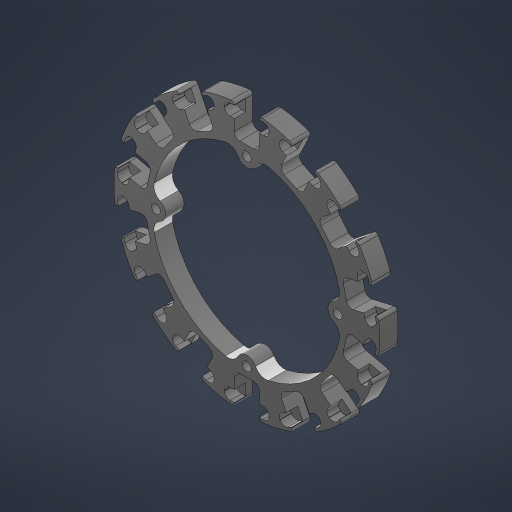
# Autodesk Inventor part: Wheel_Flame
Saved by Autodesk Inventor 2024.2 (Build 282272000, 272)
## iProperties
Created: 2023-12-20
Part Number: Wheel_Flame
Material: 一般
Document SubType Name: Modeling
Designer: Hanaoka
Density: 1 g/cm^3
Appearance: 黒
Author: Hanaoka
Autodesk Inventor part; units mm, degrees
ref_plane "YZ Plane" through (0, 0, 0) normal (1, 0, 0) x (0, 1, 0)
ref_plane "XZ Plane" through (0, 0, 0) normal (0, 1, 0) x (-1, 0, 0)
ref_plane "XY Plane" through (0, 0, 0) normal (0, 0, 1) x (1, 0, 0)
sketch "スケッチ1" plane through (0, 0, 0) normal (0, 0, 1) x (1, 0, 0)
  circle A0 centre (0, 0) radius 25 construction
  line L0 (-2.25, 24.8985) -> (-2.25, 19)
  line L1 (-1.25, 18) -> (1.25, 18)
  line L2 (2.25, 19) -> (2.25, 24.8985)
  line L3 (0, 25) -> (0, 18) construction
  line L4 (-2.25, 23.025) -> (-3, 23.025)
  line L5 (-4, 22.025) -> (-4, 21.975)
  line L6 (-3, 20.975) -> (-2.25, 20.975)
  line L7 (2.25, 23.025) -> (3, 23.025)
  line L8 (4, 22.025) -> (4, 21.975)
  line L9 (3, 20.975) -> (2.25, 20.975)
  arc A1 (-3, 23.025) -> (-4, 22.025) centre (-3, 22.025) ccw
  arc A2 (-4, 21.975) -> (-3, 20.975) centre (-3, 21.975) ccw
  arc A3 (4, 22.025) -> (3, 23.025) centre (3, 22.025) ccw
  arc A4 (3, 20.975) -> (4, 21.975) centre (3, 21.975) ccw
  arc A5 (-2.25, 19) -> (-1.25, 18) centre (-1.25, 19) ccw
  arc A6 (1.25, 18) -> (2.25, 19) centre (1.25, 19) ccw
  arc A7 (-10.271, 16.1422) -> (-8.9361, 15.6751) centre (-9.37, 16.5761) ccw
  arc A8 (-6.6837, 16.7598) -> (-6.2166, 18.0946) centre (-7.1176, 17.6608) ccw
  line L10 (-8.9361, 15.6751) -> (-6.6837, 16.7598)
  line L11 (-6.3978, 20.1995) -> (-7.0735, 19.8741)
  arc A9 (-6.3978, 20.1995) -> (-5.9307, 21.5343) centre (-6.8317, 21.1004) ccw
  line L12 (-5.9524, 21.5794) -> (-5.9307, 21.5343)
  arc A10 (-5.9524, 21.5794) -> (-7.2873, 22.0465) centre (-6.8534, 21.1455) ccw
  line L13 (-7.963, 21.721) -> (-7.2873, 22.0465)
  line L14 (-11.8036, 17.5962) -> (-11.1279, 17.9216)
  line L15 (-6.2166, 18.0946) -> (-8.7759, 23.4091)
  line L16 (-10.8471, 22.5242) -> (-7.8099, 16.2174) construction
  line L17 (-12.8303, 21.4566) -> (-10.271, 16.1422)
  arc A11 (-13.1385, 18.0633) -> (-11.8036, 17.5962) centre (-12.2375, 18.4971) ccw
  line L18 (-12.0174, 19.7686) -> (-12.6931, 19.4432)
  line L19 (-13.1602, 18.1083) -> (-13.1385, 18.0633)
  arc A12 (-12.6931, 19.4432) -> (-13.1602, 18.1083) centre (-12.2592, 18.5422) ccw
  arc A13 (-16.2577, 10.0872) -> (-14.8523, 10.2455) centre (-15.6342, 10.869) ccw
  arc A14 (-13.2936, 12.2001) -> (-13.4519, 13.6054) centre (-14.0754, 12.8236) ccw
  line L20 (-14.8523, 10.2455) -> (-13.2936, 12.2001)
  line L21 (-14.5284, 15.4232) -> (-14.9961, 14.8368)
  arc A15 (-14.5284, 15.4232) -> (-14.6868, 16.8285) centre (-15.3103, 16.0467) ccw
  line L22 (-14.7259, 16.8597) -> (-14.6868, 16.8285)
  arc A16 (-14.7259, 16.8597) -> (-16.1312, 16.7013) centre (-15.3494, 16.0779) ccw
  line L23 (-16.5988, 16.115) -> (-16.1312, 16.7013)
  line L24 (-18.2694, 10.7322) -> (-17.8018, 11.3186)
  line L25 (-13.4519, 13.6054) -> (-18.0636, 17.2831)
  line L26 (-19.5458, 15.5872) -> (-14.073, 11.2228) construction
  line L27 (-20.8693, 13.7649) -> (-16.2577, 10.0872)
  arc A17 (-19.6747, 10.5739) -> (-18.2694, 10.7322) centre (-19.0512, 11.3557) ccw
  line L28 (-19.4045, 12.5967) -> (-19.8721, 12.0104)
  line L29 (-19.7138, 10.605) -> (-19.6747, 10.5739)
  arc A18 (-19.8721, 12.0104) -> (-19.7138, 10.605) centre (-19.0903, 11.3869) ccw
  arc A19 (-19.0243, 2.0343) -> (-17.8269, 2.7867) centre (-18.8018, 3.0092) ccw
  arc A20 (-17.2706, 5.224) -> (-18.023, 6.4215) centre (-18.2455, 5.4466) ccw
  line L30 (-17.8269, 2.7867) -> (-17.2706, 5.224)
  line L31 (-19.7816, 7.5922) -> (-19.9484, 6.861)
  arc A21 (-19.7816, 7.5922) -> (-20.534, 8.7896) centre (-20.7565, 7.8147) ccw
  line L32 (-20.5827, 8.8007) -> (-20.534, 8.7896)
  arc A22 (-20.5827, 8.8007) -> (-21.7802, 8.0483) centre (-20.8052, 7.8258) ccw
  line L33 (-21.947, 7.3171) -> (-21.7802, 8.0483)
  line L34 (-21.1167, 1.7426) -> (-20.9498, 2.4738)
  line L35 (-18.023, 6.4215) -> (-23.7736, 7.734)
  line L36 (-24.3732, 5.563) -> (-17.5487, 4.0054) construction
  line L37 (-24.775, 3.3469) -> (-19.0243, 2.0343)
  arc A23 (-22.3141, 0.9902) -> (-21.1167, 1.7426) centre (-22.0916, 1.9651) ccw
  line L38 (-22.9484, 2.93) -> (-23.1153, 2.1988)
  line L39 (-22.3629, 1.0013) -> (-22.3141, 0.9902)
  arc A24 (-23.1153, 2.1988) -> (-22.3629, 1.0013) centre (-22.1404, 1.9762) ccw
  arc A25 (-18.023, -6.4215) -> (-17.2706, -5.224) centre (-18.2455, -5.4466) ccw
  arc A26 (-17.8269, -2.7867) -> (-19.0243, -2.0343) centre (-18.8018, -3.0092) ccw
  line L40 (-17.2706, -5.224) -> (-17.8269, -2.7867)
  line L41 (-21.1167, -1.7426) -> (-20.9498, -2.4738)
  arc A27 (-21.1167, -1.7426) -> (-22.3141, -0.9902) centre (-22.0916, -1.9651) ccw
  line L42 (-22.3629, -1.0013) -> (-22.3141, -0.9902)
  arc A28 (-22.3629, -1.0013) -> (-23.1153, -2.1988) centre (-22.1404, -1.9762) ccw
  line L43 (-22.9484, -2.93) -> (-23.1153, -2.1988)
  line L44 (-19.7816, -7.5922) -> (-19.9484, -6.861)
  line L45 (-19.0243, -2.0343) -> (-24.775, -3.3469)
  line L46 (-24.3732, -5.563) -> (-17.5487, -4.0054) construction
  line L47 (-23.7736, -7.734) -> (-18.023, -6.4215)
  arc A29 (-20.534, -8.7896) -> (-19.7816, -7.5922) centre (-20.7565, -7.8147) ccw
  line L48 (-21.947, -7.3171) -> (-21.7802, -8.0483)
  line L49 (-20.5827, -8.8007) -> (-20.534, -8.7896)
  arc A30 (-21.7802, -8.0483) -> (-20.5827, -8.8007) centre (-20.8052, -7.8258) ccw
  arc A31 (-13.4519, -13.6054) -> (-13.2936, -12.2001) centre (-14.0754, -12.8236) ccw
  arc A32 (-14.8523, -10.2455) -> (-16.2577, -10.0872) centre (-15.6342, -10.869) ccw
  line L50 (-13.2936, -12.2001) -> (-14.8523, -10.2455)
  line L51 (-18.2694, -10.7322) -> (-17.8018, -11.3186)
  arc A33 (-18.2694, -10.7322) -> (-19.6747, -10.5739) centre (-19.0512, -11.3557) ccw
  line L52 (-19.7138, -10.605) -> (-19.6747, -10.5739)
  arc A34 (-19.7138, -10.605) -> (-19.8721, -12.0104) centre (-19.0903, -11.3869) ccw
  line L53 (-19.4045, -12.5967) -> (-19.8721, -12.0104)
  line L54 (-14.5284, -15.4232) -> (-14.9961, -14.8368)
  line L55 (-16.2577, -10.0872) -> (-20.8693, -13.7649)
  line L56 (-19.5458, -15.5872) -> (-14.073, -11.2228) construction
  line L57 (-18.0636, -17.2831) -> (-13.4519, -13.6054)
  arc A35 (-14.6868, -16.8285) -> (-14.5284, -15.4232) centre (-15.3103, -16.0467) ccw
  line L58 (-16.5988, -16.115) -> (-16.1312, -16.7013)
  line L59 (-14.7259, -16.8597) -> (-14.6868, -16.8285)
  arc A36 (-16.1312, -16.7013) -> (-14.7259, -16.8597) centre (-15.3494, -16.0779) ccw
  arc A37 (-6.2166, -18.0946) -> (-6.6837, -16.7598) centre (-7.1176, -17.6608) ccw
  arc A38 (-8.9361, -15.6751) -> (-10.271, -16.1422) centre (-9.37, -16.5761) ccw
  line L60 (-6.6837, -16.7598) -> (-8.9361, -15.6751)
  line L61 (-11.8036, -17.5962) -> (-11.1279, -17.9216)
  arc A39 (-11.8036, -17.5962) -> (-13.1385, -18.0633) centre (-12.2375, -18.4971) ccw
  line L62 (-13.1602, -18.1083) -> (-13.1385, -18.0633)
  arc A40 (-13.1602, -18.1083) -> (-12.6931, -19.4432) centre (-12.2592, -18.5422) ccw
  line L63 (-12.0174, -19.7686) -> (-12.6931, -19.4432)
  line L64 (-6.3978, -20.1995) -> (-7.0735, -19.8741)
  line L65 (-10.271, -16.1422) -> (-12.8303, -21.4566)
  line L66 (-10.8471, -22.5242) -> (-7.8099, -16.2174) construction
  line L67 (-8.7759, -23.4091) -> (-6.2166, -18.0946)
  arc A41 (-5.9307, -21.5343) -> (-6.3978, -20.1995) centre (-6.8317, -21.1004) ccw
  line L68 (-7.963, -21.721) -> (-7.2873, -22.0465)
  line L69 (-5.9524, -21.5794) -> (-5.9307, -21.5343)
  arc A42 (-7.2873, -22.0465) -> (-5.9524, -21.5794) centre (-6.8534, -21.1455) ccw
  arc A43 (2.25, -19) -> (1.25, -18) centre (1.25, -19) ccw
  arc A44 (-1.25, -18) -> (-2.25, -19) centre (-1.25, -19) ccw
  line L70 (1.25, -18) -> (-1.25, -18)
  line L71 (-3, -20.975) -> (-2.25, -20.975)
  arc A45 (-3, -20.975) -> (-4, -21.975) centre (-3, -21.975) ccw
  line L72 (-4, -22.025) -> (-4, -21.975)
  arc A46 (-4, -22.025) -> (-3, -23.025) centre (-3, -22.025) ccw
  line L73 (-2.25, -23.025) -> (-3, -23.025)
  line L74 (3, -20.975) -> (2.25, -20.975)
  line L75 (-2.25, -19) -> (-2.25, -24.8985)
  line L76 (0, -25) -> (0, -18) construction
  line L77 (2.25, -24.8985) -> (2.25, -19)
  arc A47 (4, -21.975) -> (3, -20.975) centre (3, -21.975) ccw
  line L78 (2.25, -23.025) -> (3, -23.025)
  line L79 (4, -22.025) -> (4, -21.975)
  arc A48 (3, -23.025) -> (4, -22.025) centre (3, -22.025) ccw
  arc A49 (10.271, -16.1422) -> (8.9361, -15.6751) centre (9.37, -16.5761) ccw
  arc A50 (6.6837, -16.7598) -> (6.2166, -18.0946) centre (7.1176, -17.6608) ccw
  line L80 (8.9361, -15.6751) -> (6.6837, -16.7598)
  line L81 (6.3978, -20.1995) -> (7.0735, -19.8741)
  arc A51 (6.3978, -20.1995) -> (5.9307, -21.5343) centre (6.8317, -21.1004) ccw
  line L82 (5.9524, -21.5794) -> (5.9307, -21.5343)
  arc A52 (5.9524, -21.5794) -> (7.2873, -22.0465) centre (6.8534, -21.1455) ccw
  line L83 (7.963, -21.721) -> (7.2873, -22.0465)
  line L84 (11.8036, -17.5962) -> (11.1279, -17.9216)
  line L85 (6.2166, -18.0946) -> (8.7759, -23.4091)
  line L86 (10.8471, -22.5242) -> (7.8099, -16.2174) construction
  line L87 (12.8303, -21.4566) -> (10.271, -16.1422)
  arc A53 (13.1385, -18.0633) -> (11.8036, -17.5962) centre (12.2375, -18.4971) ccw
  line L88 (12.0174, -19.7686) -> (12.6931, -19.4432)
  line L89 (13.1602, -18.1083) -> (13.1385, -18.0633)
  arc A54 (12.6931, -19.4432) -> (13.1602, -18.1083) centre (12.2592, -18.5422) ccw
  arc A55 (16.2577, -10.0872) -> (14.8523, -10.2455) centre (15.6342, -10.869) ccw
  arc A56 (13.2936, -12.2001) -> (13.4519, -13.6054) centre (14.0754, -12.8236) ccw
  line L90 (14.8523, -10.2455) -> (13.2936, -12.2001)
  line L91 (14.5284, -15.4232) -> (14.9961, -14.8368)
  arc A57 (14.5284, -15.4232) -> (14.6868, -16.8285) centre (15.3103, -16.0467) ccw
  line L92 (14.7259, -16.8597) -> (14.6868, -16.8285)
  arc A58 (14.7259, -16.8597) -> (16.1312, -16.7013) centre (15.3494, -16.0779) ccw
  line L93 (16.5988, -16.115) -> (16.1312, -16.7013)
  line L94 (18.2694, -10.7322) -> (17.8018, -11.3186)
  line L95 (13.4519, -13.6054) -> (18.0636, -17.2831)
  line L96 (19.5458, -15.5872) -> (14.073, -11.2228) construction
  line L97 (20.8693, -13.7649) -> (16.2577, -10.0872)
  arc A59 (19.6747, -10.5739) -> (18.2694, -10.7322) centre (19.0512, -11.3557) ccw
  line L98 (19.4045, -12.5967) -> (19.8721, -12.0104)
  line L99 (19.7138, -10.605) -> (19.6747, -10.5739)
  arc A60 (19.8721, -12.0104) -> (19.7138, -10.605) centre (19.0903, -11.3869) ccw
  arc A61 (19.0243, -2.0343) -> (17.8269, -2.7867) centre (18.8018, -3.0092) ccw
  arc A62 (17.2706, -5.224) -> (18.023, -6.4215) centre (18.2455, -5.4466) ccw
  line L100 (17.8269, -2.7867) -> (17.2706, -5.224)
  line L101 (19.7816, -7.5922) -> (19.9484, -6.861)
  arc A63 (19.7816, -7.5922) -> (20.534, -8.7896) centre (20.7565, -7.8147) ccw
  line L102 (20.5827, -8.8007) -> (20.534, -8.7896)
  arc A64 (20.5827, -8.8007) -> (21.7802, -8.0483) centre (20.8052, -7.8258) ccw
  line L103 (21.947, -7.3171) -> (21.7802, -8.0483)
  line L104 (21.1167, -1.7426) -> (20.9498, -2.4738)
  line L105 (18.023, -6.4215) -> (23.7736, -7.734)
  line L106 (24.3732, -5.563) -> (17.5487, -4.0054) construction
  line L107 (24.775, -3.3469) -> (19.0243, -2.0343)
  arc A65 (22.3141, -0.9902) -> (21.1167, -1.7426) centre (22.0916, -1.9651) ccw
  line L108 (22.9484, -2.93) -> (23.1153, -2.1988)
  line L109 (22.3629, -1.0013) -> (22.3141, -0.9902)
  arc A66 (23.1153, -2.1988) -> (22.3629, -1.0013) centre (22.1404, -1.9762) ccw
  arc A67 (18.023, 6.4215) -> (17.2706, 5.224) centre (18.2455, 5.4466) ccw
  arc A68 (17.8269, 2.7867) -> (19.0243, 2.0343) centre (18.8018, 3.0092) ccw
  line L110 (17.2706, 5.224) -> (17.8269, 2.7867)
  line L111 (21.1167, 1.7426) -> (20.9498, 2.4738)
  arc A69 (21.1167, 1.7426) -> (22.3141, 0.9902) centre (22.0916, 1.9651) ccw
  line L112 (22.3629, 1.0013) -> (22.3141, 0.9902)
  arc A70 (22.3629, 1.0013) -> (23.1153, 2.1988) centre (22.1404, 1.9762) ccw
  line L113 (22.9484, 2.93) -> (23.1153, 2.1988)
  line L114 (19.7816, 7.5922) -> (19.9484, 6.861)
  line L115 (19.0243, 2.0343) -> (24.775, 3.3469)
  line L116 (24.3732, 5.563) -> (17.5487, 4.0054) construction
  line L117 (23.7736, 7.734) -> (18.023, 6.4215)
  arc A71 (20.534, 8.7896) -> (19.7816, 7.5922) centre (20.7565, 7.8147) ccw
  line L118 (21.947, 7.3171) -> (21.7802, 8.0483)
  line L119 (20.5827, 8.8007) -> (20.534, 8.7896)
  arc A72 (21.7802, 8.0483) -> (20.5827, 8.8007) centre (20.8052, 7.8258) ccw
  arc A73 (13.4519, 13.6054) -> (13.2936, 12.2001) centre (14.0754, 12.8236) ccw
  arc A74 (14.8523, 10.2455) -> (16.2577, 10.0872) centre (15.6342, 10.869) ccw
  line L120 (13.2936, 12.2001) -> (14.8523, 10.2455)
  line L121 (18.2694, 10.7322) -> (17.8018, 11.3186)
  arc A75 (18.2694, 10.7322) -> (19.6747, 10.5739) centre (19.0512, 11.3557) ccw
  line L122 (19.7138, 10.605) -> (19.6747, 10.5739)
  arc A76 (19.7138, 10.605) -> (19.8721, 12.0104) centre (19.0903, 11.3869) ccw
  line L123 (19.4045, 12.5967) -> (19.8721, 12.0104)
  line L124 (14.5284, 15.4232) -> (14.9961, 14.8368)
  line L125 (16.2577, 10.0872) -> (20.8693, 13.7649)
  line L126 (19.5458, 15.5872) -> (14.073, 11.2228) construction
  line L127 (18.0636, 17.2831) -> (13.4519, 13.6054)
  arc A77 (14.6868, 16.8285) -> (14.5284, 15.4232) centre (15.3103, 16.0467) ccw
  line L128 (16.5988, 16.115) -> (16.1312, 16.7013)
  line L129 (14.7259, 16.8597) -> (14.6868, 16.8285)
  arc A78 (16.1312, 16.7013) -> (14.7259, 16.8597) centre (15.3494, 16.0779) ccw
  arc A79 (6.2166, 18.0946) -> (6.6837, 16.7598) centre (7.1176, 17.6608) ccw
  arc A80 (8.9361, 15.6751) -> (10.271, 16.1422) centre (9.37, 16.5761) ccw
  line L130 (6.6837, 16.7598) -> (8.9361, 15.6751)
  line L131 (11.8036, 17.5962) -> (11.1279, 17.9216)
  arc A81 (11.8036, 17.5962) -> (13.1385, 18.0633) centre (12.2375, 18.4971) ccw
  line L132 (13.1602, 18.1083) -> (13.1385, 18.0633)
  arc A82 (13.1602, 18.1083) -> (12.6931, 19.4432) centre (12.2592, 18.5422) ccw
  line L133 (12.0174, 19.7686) -> (12.6931, 19.4432)
  line L134 (6.3978, 20.1995) -> (7.0735, 19.8741)
  line L135 (10.271, 16.1422) -> (12.8303, 21.4566)
  line L136 (10.8471, 22.5242) -> (7.8099, 16.2174) construction
  line L137 (8.7759, 23.4091) -> (6.2166, 18.0946)
  arc A83 (5.9307, 21.5343) -> (6.3978, 20.1995) centre (6.8317, 21.1004) ccw
  line L138 (7.963, 21.721) -> (7.2873, 22.0465)
  line L139 (5.9524, 21.5794) -> (5.9307, 21.5343)
  arc A84 (7.2873, 22.0465) -> (5.9524, 21.5794) centre (6.8534, 21.1455) ccw
  circle A85 centre (0, 0) radius 23.75
  circle A86 centre (0, 0) radius 17
  circle A87 centre (0, 0) radius 2
  line L140 (-2, -3.5) -> (2, -3.5)
  line L141 (3.5, -2) -> (3.5, 2)
  line L142 (2, 3.5) -> (-2, 3.5)
  line L143 (-3.5, 2) -> (-3.5, -2)
  line L144 (-3.5, -3.5) -> (3.5, 3.5) construction
  line L145 (3.5, -3.5) -> (-3.5, 3.5) construction
  arc A88 (-2, 3.5) -> (-3.5, 2) centre (-2, 2) ccw
  arc A89 (-3.5, -2) -> (-2, -3.5) centre (-2, -2) ccw
  arc A90 (2, -3.5) -> (3.5, -2) centre (2, -2) ccw
  arc A91 (3.5, 2) -> (2, 3.5) centre (2, 2) ccw
  line L146 (-1.75, 16.9097) -> (-1.75, 3.5)
  line L147 (1.75, 3.5) -> (1.75, 16.9097)
  circle A92 centre (0, 16.25) radius 0.8
  line L148 (0, -35) -> (0, 35) projected
  circle A93 centre (0, 16.25) radius 1.75
  circle A94 centre (-16.25, 0) radius 0.8
  line L149 (-3.5, 1.75) -> (-16.9097, 1.75)
  line L150 (-16.9097, -1.75) -> (-3.5, -1.75)
  circle A95 centre (0, -16.25) radius 0.8
  line L151 (-1.75, -3.5) -> (-1.75, -16.9097)
  line L152 (1.75, -16.9097) -> (1.75, -3.5)
  circle A96 centre (16.25, 0) radius 0.8
  line L153 (3.5, -1.75) -> (16.9097, -1.75)
  line L154 (16.9097, 1.75) -> (3.5, 1.75)
  circle A97 centre (-16.25, 0) radius 1.75
  circle A98 centre (0, -16.25) radius 1.75
  circle A99 centre (16.25, 0) radius 1.75
  line L155 (-1.3229, 1.5) -> (1.3229, 1.5)
  circle A100 centre (0, 0) radius 14.5
  point P0 (-2.25, 18)
  point P1 (2.25, 18)
  point P2 (4, 23.025)
  point P3 (4, 20.975)
  point P4 (-4, 22)
  point P5 (-9.8371, 15.2412)
  point P6 (-5.7827, 17.1937)
  point P7 (-5.4968, 20.6334)
  point P8 (-6.3863, 22.4803)
  point P9 (-13.1493, 18.0858)
  point P10 (-15.4758, 9.4637)
  point P11 (-12.6701, 12.9819)
  point P12 (-13.905, 16.205)
  point P13 (-15.5077, 17.4832)
  point P14 (-19.6943, 10.5894)
  point P15 (-18.0494, 1.8118)
  point P16 (-17.048, 6.199)
  point P17 (-19.559, 8.5671)
  point P18 (-21.5576, 9.0233)
  point P19 (-22.3385, 0.9957)
  point P20 (-17.048, -6.199)
  point P21 (-18.0494, -1.8118)
  point P22 (-21.3392, -0.7677)
  point P23 (-23.3378, -1.2238)
  point P24 (-20.5583, -8.7952)
  point P25 (-12.6701, -12.9819)
  point P26 (-15.4758, -9.4637)
  point P27 (-18.8929, -9.9504)
  point P28 (-20.4956, -11.2285)
  point P29 (-14.7063, -16.8441)
  point P30 (-5.7827, -17.1937)
  point P31 (-9.8371, -15.2412)
  point P32 (-12.7046, -17.1623)
  point P33 (-13.594, -19.0093)
  point P34 (-5.9416, -21.5569)
  point P35 (2.25, -18)
  point P36 (-2.25, -18)
  point P37 (-4, -20.975)
  point P38 (-4, -23.025)
  point P39 (4, -22)
  point P40 (9.8371, -15.2412)
  point P41 (5.7827, -17.1937)
  point P42 (5.4968, -20.6334)
  point P43 (6.3863, -22.4803)
  point P44 (13.1493, -18.0858)
  point P45 (15.4758, -9.4637)
  point P46 (12.6701, -12.9819)
  point P47 (13.905, -16.205)
  point P48 (15.5077, -17.4832)
  point P49 (19.6943, -10.5894)
  point P50 (18.0494, -1.8118)
  point P51 (17.048, -6.199)
  point P52 (19.559, -8.5671)
  point P53 (21.5576, -9.0233)
  point P54 (22.3385, -0.9957)
  point P55 (17.048, 6.199)
  point P56 (18.0494, 1.8118)
  point P57 (21.3392, 0.7677)
  point P58 (23.3378, 1.2238)
  point P59 (20.5583, 8.7952)
  point P60 (12.6701, 12.9819)
  point P61 (15.4758, 9.4637)
  point P62 (18.8929, 9.9504)
  point P63 (20.4956, 11.2285)
  point P64 (14.7063, 16.8441)
  point P65 (5.7827, 17.1937)
  point P66 (9.8371, 15.2412)
  point P67 (12.7046, 17.1623)
  point P68 (13.594, 19.0093)
  point P69 (5.9416, 21.5569)
  point P70 (-2.25, 23.6432)
  point P71 (-8.2312, 22.278)
  point P72 (-12.2856, 20.3255)
  point P73 (-17.0821, 16.5004)
  point P74 (-19.8878, 12.9822)
  point P75 (-22.5497, 7.4547)
  point P76 (-23.5511, 3.0675)
  point P77 (-23.5511, -3.0675)
  point P78 (-22.5497, -7.4547)
  point P79 (-19.8878, -12.9822)
  point P80 (-17.0821, -16.5004)
  point P81 (-12.2856, -20.3255)
  point P82 (-8.2312, -22.278)
  point P83 (-2.25, -23.6432)
  point P84 (2.25, -23.6432)
  point P85 (8.2312, -22.278)
  point P86 (12.2856, -20.3255)
  point P87 (17.0821, -16.5004)
  point P88 (19.8878, -12.9822)
  point P89 (22.5497, -7.4547)
  point P90 (23.5511, -3.0675)
  point P91 (23.5511, 3.0675)
  point P92 (22.5497, 7.4547)
  point P93 (19.8878, 12.9822)
  point P94 (17.0821, 16.5004)
  point P95 (12.2856, 20.3255)
  point P96 (8.2312, 22.278)
  point P97 (2.25, 23.6432)
  point P98 (1.75, 16.25)
  point P99 (16.25, 1.75)
  point P100 (16.25, -1.75)
  point P101 (1.75, -16.9097)
  point P102 (1.75, -16.25)
  point P103 (-1.75, -16.25)
  point P104 (-16.9097, -1.75)
  point P105 (-16.25, -1.75)
  point P106 (-16.25, 1.75)
  point P107 (-16.9097, 1.75)
  point P108 (-1.75, 16.25)
  point P109 (1.75, 14.394)
  point P110 (14.394, 1.75)
  point P111 (14.394, -1.75)
  point P112 (1.75, -14.394)
  point P113 (-1.75, -14.394)
  point P114 (-14.394, -1.75)
  point P115 (-14.394, 1.75)
  point P116 (-1.75, 14.394)
  point P117 (0, -14.5)
  point P118 (14.5, 0)
  point P119 (-14.5, 0)
  point P120 (0, 14.5)
  dimension "d14" = 47.5
  dimension "d0" = 50
  dimension "d1" = 4.5
  dimension "d2" = 1
  dimension "d5" = 2.05
  dimension "d6" = 8
  dimension "d7" = 1
  dimension "d8" = 7
  dimension "d9" = 3
  dimension "d12" = 360
  dimension "d19" = 34
  dimension "d20" = 4
  dimension "d21" = 1.5
  dimension "d22" = 4
  dimension "d23" = 3.5
  dimension "d24" = 1.6
  dimension "d25" = 3.5
  dimension "d28" = 360
  dimension "d32" = 360
  dimension "d35" = 1.5
  constraints: 310 end point, 235 point on line, 183 point on circle, 100 centre point, 22 tangent, 7 equal radius, 6 coincident, 6 perpendicular, 5 parallel, 4 equal length, 4 midpoint, 3 horizontal, 1 vertical, 703 other
  measures "d0" diameter of A0
  measures "d1" distance of point (-2.25, 18) point (2.25, 18)
  measures "d2" radius of A1
  measures "d5" distance between parallel lines of L6 L4
  measures "d6" distance between parallel lines of L8 L5
  measures "d7" radius of A5
  measures "d8" distance of L3.start L3.end
  measures "d9" vertical distance of point (-4, 22) L3.start
  measures "d19" diameter of A86
  measures "d20" diameter of A87
  measures "d21" radius of A88
  measures "d22" distance of L142.start L142.end
  measures "d23" distance between parallel lines of L147 L146
  measures "d24" diameter of A92
  measures "d25" diameter of A93
  measures "d35" distance from line of A0.centre L155
extrude "押し出し1" add sketch "スケッチ1" along normal blind 2.05 contours L4 A1 L5 A2 L6 L0 A5 L1 A93 A86 A97 A98 L70 A44 L75 L71 A45 L72 A46 L73 A85 L67 L68 A42 L69 A41 L64 A37 L60 A38 L65 L61 A39 L62 A40 L63 L57 L58 A36 L59 A35 L54 A31 L50 A32 L55 L51 A33 L52 A34 L53 L47 L48 A30 L49 A29 L44 A25 L40 A26 L45 L41 A27 L42 A28 L43 L37 L38 A24 L39 A23 L34 A19 L30 A20 L35 L31 A21 L32 A22 L33 L27 L28 A18 L29 A17 L24 A13 L20 A14 L25 L21 A15 L22 A16 L23 L17 L18 A12 L19 A11 L14 A7 L10 A8 L15 L11 A9 L12 A10 L13 | A85 L137 L138 A84 L139 A83 L134 A79 L130 A80 L135 L131 A81 L132 A82 L133 L127 L128 A78 L129 A77 L124 A73 L120 A74 L125 L121 A75 L122 A76 L123 L117 L118 A72 L119 A71 L114 A67 L110 A68 L115 L111 A69 L112 A70 L113 L107 L108 A66 L109 A65 L104 A61 L100 A62 L105 L101 A63 L102 A64 L103 L97 L98 A60 L99 A59 L94 A55 L90 A56 L95 L91 A57 L92 A58 L93 L87 L88 A54 L89 A53 L84 A49 L80 A50 L85 L81 A51 L82 A52 L83 L77 L78 A48 L79 A47 L74 A43 L70 A98 A86 A99 A93 L1 A6 L2 L9 A4 L8 A3 L7 | A93 A86 A92 L148 | L148 A92 A86 A93 | A93 L148 A92 A86 | A86 L147 A93 | A93 L146 A86 | A86 A92 L148 A93 | A86 A99 L154 | L149 A97 A86 | A99 A86 A96 | A86 A96 A99 | A97 A86 A94 | A86 A94 A97 | A97 L150 A86 | A86 L153 A99 | L151 A98 A86 | A86 A98 L152 | A98 A86 A95 L148 | L148 A95 A86 A98 | A86 A95 L148 A98 | A98 L148 A95 A86
extrude "押し出し2" add sketch "スケッチ1" against normal blind 1.25 contours L4 A1 L5 A2 L6 L0 A5 L1 A93 A86 A97 A98 L70 A44 L75 L71 A45 L72 A46 L73 A85 L67 L68 A42 L69 A41 L64 A37 L60 A38 L65 L61 A39 L62 A40 L63 L57 L58 A36 L59 A35 L54 A31 L50 A32 L55 L51 A33 L52 A34 L53 L47 L48 A30 L49 A29 L44 A25 L40 A26 L45 L41 A27 L42 A28 L43 L37 L38 A24 L39 A23 L34 A19 L30 A20 L35 L31 A21 L32 A22 L33 L27 L28 A18 L29 A17 L24 A13 L20 A14 L25 L21 A15 L22 A16 L23 L17 L18 A12 L19 A11 L14 A7 L10 A8 L15 L11 A9 L12 A10 L13 | L0 L6 A2 L5 A1 L4 | A85 L137 L138 A84 L139 A83 L134 A79 L130 A80 L135 L131 A81 L132 A82 L133 L127 L128 A78 L129 A77 L124 A73 L120 A74 L125 L121 A75 L122 A76 L123 L117 L118 A72 L119 A71 L114 A67 L110 A68 L115 L111 A69 L112 A70 L113 L107 L108 A66 L109 A65 L104 A61 L100 A62 L105 L101 A63 L102 A64 L103 L97 L98 A60 L99 A59 L94 A55 L90 A56 L95 L91 A57 L92 A58 L93 L87 L88 A54 L89 A53 L84 A49 L80 A50 L85 L81 A51 L82 A52 L83 L77 L78 A48 L79 A47 L74 A43 L70 A98 A86 A99 A93 L1 A6 L2 L9 A4 L8 A3 L7 | A93 A86 A92 L148 | L148 A92 A86 A93 | L13 A10 L12 A9 L11 L15 | L7 A3 L8 A4 L9 L2 | A93 L148 A92 A86 | A86 L147 A93 | A93 L146 A86 | A86 A92 L148 A93 | L17 L14 A11 L19 A12 L18 | L137 L134 A83 L139 A84 L138 | L23 A16 L22 A15 L21 L25 | L133 A82 L132 A81 L131 L135 | A86 A99 L154 | L149 A97 A86 | L27 L24 A17 L29 A18 L28 | L127 L124 A77 L129 A78 L128 | A99 A86 A96 | A86 A96 A99 | A97 A86 A94 | A86 A94 A97 | L33 A22 L32 A21 L31 L35 | L123 A76 L122 A75 L121 L125 | A97 L150 A86 | L37 L34 A23 L39 A24 L38 | L117 L114 A71 L119 A72 L118 | A86 L153 A99 | L43 A28 L42 A27 L41 L45 | L113 A70 L112 A69 L111 L115 | L151 A98 A86 | L47 L44 A29 L49 A30 L48 | A86 A98 L152 | A98 A86 A95 L148 | L148 A95 A86 A98 | A86 A95 L148 A98 | L53 A34 L52 A33 L51 L55 | L107 L104 A65 L109 A66 L108 | A98 L148 A95 A86 | L57 L54 A35 L59 A36 L58 | L103 A64 L102 A63 L101 L105 | L63 A40 L62 A39 L61 L65 | L97 L94 A59 L99 A60 L98 | L67 L64 A41 L69 A42 L68 | L93 A58 L92 A57 L91 L95 | L74 A47 L79 A48 L78 L77 | L75 L73 A46 L72 A45 L71 | L87 L84 A53 L89 A54 L88 | L83 A52 L82 A51 L81 L85
fillet "フィレット2" radius 0.5 28 edges at (-2.25, 23.6432, 0.4) (-8.2312, 22.278, 0.4) (-12.2856, 20.3255, 0.4) (-17.0821, 16.5004, 0.4) (-19.8878, 12.9822, 0.4) (-22.5497, 7.4547, 0.4) (-23.5511, 3.0675, 0.4) (-23.5511, -3.0675, 0.4) (-22.5497, -7.4547, 0.4) (-19.8878, -12.9822, 0.4) (-17.0821, -16.5004, 0.4) (-12.2856, -20.3255, 0.4) (-8.2312, -22.278, 0.4) (-2.25, -23.6432, 0.4) (2.25, -23.6432, 0.4) (8.2312, -22.278, 0.4) (12.2856, -20.3255, 0.4) (17.0821, -16.5004, 0.4) (22.5497, -7.4547, 0.4) (23.5511, -3.0675, 0.4) (23.5511, 3.0675, 0.4) (22.5497, 7.4547, 0.4) (19.8878, 12.9822, 0.4) (17.0821, 16.5004, 0.4) (12.2856, 20.3255, 0.4) (8.2312, 22.278, 0.4) (2.25, 23.6432, 0.4) (19.8878, -12.9822, 0.4)
fillet "フィレット3" radius 2 8 edges at (-1.75, 16.9097, 0.4) (1.75, 16.9097, 0.4) (-16.9097, 1.75, 0.4) (-16.9097, -1.75, 0.4) (-1.75, -16.9097, 0.4) (1.75, -16.9097, 0.4) (16.9097, 1.75, 0.4) (16.9097, -1.75, 0.4)
